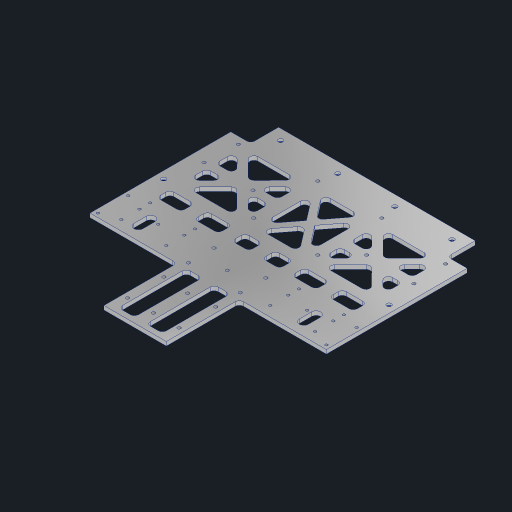
# Autodesk Inventor part: base
Saved by Autodesk Inventor 2023 (Build 270158000, 158)
## iProperties
Created: 2024-04-10
Part Number: base
Material: Aluminum 6061
Document SubType Name: Modeling
Designer: szymo
Density: 2.7 g/cm^3
Appearance: Aluminum - Flat
Mass: 138.037 g
Surface Area: 408.524 cm^2
Volume: 51.1249 cm^3
Author: szymo
Autodesk Inventor part; units mm, degrees
ref_plane "YZ Plane" through (0, 0, 0) normal (1, 0, 0) x (0, 1, 0)
ref_plane "XZ Plane" through (0, 0, 0) normal (0, 1, 0) x (-1, 0, 0)
ref_plane "XY Plane" through (0, 0, 0) normal (0, 0, 1) x (1, 0, 0)
sketch "Sketch2" plane through (0, 0, 0) normal (0, 1, 0) x (-1, 0, 0)
  line L0 (-89, 99) -> (89, 99)
  line L1 (89, 99) -> (89, -99)
  line L2 (89, -99) -> (-89, -99)
  line L3 (-89, -99) -> (-89, 99)
  line L4 (-89, 99) -> (89, -99) construction
  line L5 (89, 99) -> (-89, -99) construction
  line L6 (-89, 99) -> (89, 99)
  line L7 (89, 99) -> (89, -85)
  line L8 (89, -85) -> (-89, -85)
  line L9 (-89, -85) -> (-89, 99)
  line L10 (-4.5, 99) -> (-89, 99)
  line L11 (-89, 99) -> (-89, 42)
  line L12 (-89, 42) -> (-4.5, 42)
  line L13 (-4.5, 42) -> (-4.5, 99)
  line L14 (4.5, 99) -> (89, 99)
  line L15 (89, 99) -> (89, 42)
  line L16 (89, 42) -> (4.5, 42)
  line L17 (4.5, 42) -> (4.5, 99)
  line L18 (22.5, 77.5) -> (22.5, 66.5) projected
  line L19 (16.5, 66.5) -> (16.5, 77.5) projected
  line L20 (-22.5, 66.5) -> (-22.5, 77.5) projected
  line L21 (-16.5, 77.5) -> (-16.5, 66.5) projected
  line L22 (-23.5, 99) -> (-16.5, 99)
  line L23 (-16.5, 99) -> (-16.5, 42)
  line L24 (-16.5, 42) -> (-23.5, 42)
  line L25 (-23.5, 42) -> (-23.5, 99)
  line L26 (16.5, 99) -> (23.5, 99)
  line L27 (23.5, 99) -> (23.5, 42)
  line L28 (23.5, 42) -> (16.5, 42)
  line L29 (16.5, 42) -> (16.5, 99)
  line L30 (-89, 99) -> (89, 99)
  line L31 (89, 99) -> (89, 97)
  line L32 (89, 97) -> (-89, 97)
  line L33 (-89, 97) -> (-89, 99)
  line L34 (89, -85) -> (74, -85)
  line L35 (74, -85) -> (74, -64)
  line L36 (74, -64) -> (89, -64)
  line L37 (89, -64) -> (89, -85)
  line L38 (-89, -85) -> (-74, -85)
  line L39 (-74, -85) -> (-74, -64)
  line L40 (-74, -64) -> (-89, -64)
  line L41 (-89, -64) -> (-89, -85)
  line L42 (16.5, 97) -> (-16.5, 97)
  line L43 (-16.5, 97) -> (-16.5, 93)
  line L44 (-16.5, 93) -> (16.5, 93)
  line L45 (16.5, 93) -> (16.5, 97)
  line L46 (-84.4, -75) -> (-84.4, -71.5) projected
  line L47 (-84.4, -71.5) -> (-87, -71.5) projected
  line L48 (-87, -71.5) -> (-87, -75) projected
  line L49 (-87, -75) -> (-84.4, -75) projected
  line L50 (-79.6, -75) -> (-77, -75) projected
  line L51 (-77, -75) -> (-77, -71.5) projected
  line L52 (-77, -71.5) -> (-79.6, -71.5) projected
  line L53 (-79.6, -71.5) -> (-79.6, -75) projected
  line L54 (-75, -78) -> (-89, -78) projected
  line L55 (-89, -78) -> (-89, -63) projected
  line L56 (-89, -63) -> (-75, -63) projected
  line L57 (-75, -63) -> (-75, -78) projected
  circle A0 centre (-80.45, -67.25) radius 1.25 projected
  point P0 (0, 0)
  point P1 (4.5, 99)
  point P2 (-4.5, 99)
  point P3 (-89, 42)
  point P4 (89, 42)
  point P5 (4.5, 97)
  point P6 (-4.5, 97)
  point P7 (-16.5, 97)
  point P8 (-23.5, 97)
  point P9 (23.5, 97)
  point P10 (16.5, 98)
  point P11 (-4.5, 93)
  point P12 (4.5, 93)
  point P13 (16.5, 93)
  dimension "d8" = 178
  dimension "d9" = 198
  dimension "d10" = 14
  dimension "d11" = 84.5
  dimension "d13" = 84.5
  dimension "d17" = 9
  dimension "d18" = 2
  dimension "d19" = 15
  dimension "d20" = 21
  dimension "d21" = 15
  dimension "d22" = 21
  dimension "d75" = 55
  dimension "d76" = 55
  dimension "d77" = 7
  dimension "d78" = 7
  dimension "d79" = 4
  constraints: 84 end point, 20 parallel, 10 horizontal, 10 perpendicular, 10 point on line, 2 collinear, 2 midpoint, 5 other
  measures "d8" distance of L1.end L2.end
  measures "d9" distance of L0.end L1.end
  measures "d10" distance between parallel lines of L8 L2
  measures "d11" distance of L12.end L11.end
  measures "d13" distance of L15.end L16.end
  measures "d17" distance between parallel lines of L13 L17
  measures "d18" distance of L30.end L31.end
  measures "d19" distance of L35.end L36.end
  measures "d20" distance of L34.end L35.end
  measures "d21" distance of L40.end L39.end
  measures "d22" distance of L39.end L38.end
  measures "d75" distance between parallel lines of L32 L12
  measures "d76" distance between parallel lines of L32 L16
  measures "d77" distance between parallel lines of L23 L25
  measures "d78" distance between parallel lines of L27 L29
  measures "d79" distance of L43.end L42.end
extrude "Extrusion2" add sketch "Sketch2" along normal blind 3 contours L32 L23 L21 L12 L25 | L12 L13 L44 L17 L16 L1 L36 L35 L8 L39 L40 L57 L56 L3 | L32 L13 L44 L23 | L56 L57 L40 L3 | L32 L17 L44 L13 | L32 L29 L44 L17 | L32 L27 L16 L29 L19
fillet "Fillet5" radius 3 12 edges at (-16.5, 1.5, 42) (-4.5, 1.5, 42) (-23.5, 1.5, 42) (16.5, 1.5, 42) (-16.5, 1.5, 93) (-4.5, 1.5, 93) (4.5, 1.5, 93) (16.5, 1.5, 93) (4.5, 1.5, 42) (23.5, 1.5, 42) (74, 1.5, -64) (-74, 1.5, -64)
sketch "Sketch7" plane through (0, 3, 0) normal (0, 1, 0) x (1, 0, 0)
  circle A0 centre (78, 58.6725) radius 1.8 projected
  circle A1 centre (79, 33.8889) radius 1.8 projected
  circle A2 centre (42.5, 34.7802) radius 1.8 projected
  circle A3 centre (24.1, 64.6) radius 1.6 projected
  circle A4 centre (24.1, 16.4) radius 1.6 projected
  circle A5 centre (-24.1, 16.4) radius 1.6 projected
  circle A6 centre (-24.1, 64.6) radius 1.6 projected
  circle A7 centre (-42.5, 34.2745) radius 1.8 projected
  circle A8 centre (-79, 33.8889) radius 1.8 projected
  circle A9 centre (-78, 58.6725) radius 1.8 projected
  circle A10 centre (19.5, -18.05) radius 1.8 projected
  circle A11 centre (19.5, -37.375) radius 1.8 projected
  circle A12 centre (19.5, -55.8) radius 1.8 projected
  circle A13 centre (19.4231, -83.3077) radius 1.8 projected
  circle A14 centre (0, -83.2) radius 1.8 projected
  circle A15 centre (-19.4231, -83.3077) radius 1.8 projected
  circle A16 centre (-19.5, -55.8) radius 1.8 projected
  circle A17 centre (0, -57.55) radius 1.8 projected
  circle A18 centre (0, -27.625) radius 1.8 projected
  circle A19 centre (-19.5, -37.375) radius 1.8 projected
  circle A20 centre (-19.5, -18.05) radius 1.8 projected
  point P0 (0, 0)
  point P1 (-19.5, -83.2)
  constraints: 20 coincident
hole "Hole3" at (19.4231, 3, 83.3077) at (0, 3, 83.2) at (-19.5, 3, 83.2) at (19.5, 3, 55.8) at (0, 3, 57.55) at (-19.5, 3, 55.8) at (-19.5, 3, 37.375) at (-19.5, 3, 18.05) at (0, 3, 27.625) at (19.5, 3, 37.375) at (19.5, 3, 18.05) at (79, 3, -33.8889) at (78, 3, -58.6725) at (42.5, 3, -34.7802) at (24.1, 3, -16.4) at (-24.1, 3, -16.4) at (-24.1, 3, -64.6) at (24.1, 3, -64.6) at (-42.5, 3, -34.2745) at (-78, 3, -58.6725) at (-79, 3, -33.8889) direction (0, -1, 0) diameter 2.459 end through all thread size "M3x0.5" class "6H" standard "ISO Metric profile"
sketch "Sketch8" plane through (0, 3, 0) normal (0, 1, 0) x (1, 0, 0)
  circle A0 centre (72.95, -34.475) radius 1.45 projected
  circle A1 centre (72.95, -20.775) radius 1.45 projected
  circle A2 centre (39.125, -20.8375) radius 1.55 projected
  circle A3 centre (39.125, -34.4125) radius 1.55 projected
  circle A4 centre (-39.125, -20.8375) radius 1.55 projected
  circle A5 centre (-39.125, -34.4125) radius 1.55 projected
  circle A6 centre (-72.95, -34.475) radius 1.45 projected
  circle A7 centre (-72.95, -20.775) radius 1.45 projected
  circle A8 centre (86, -16.25) radius 2.3 projected
  circle A9 centre (86, -39) radius 2.3 projected
  circle A10 centre (86, 32.8889) radius 2.3 projected
  line L0 (89, -42) -> (83, -42) projected
  line L1 (89, 35.8889) -> (89, -42) projected
  line L2 (89, 35.8889) -> (83, 35.8889) projected
  line L3 (83, 29.8889) -> (83, 35.8889) projected
  line L4 (83, 29.8889) -> (87.4, 29.8889) projected
  line L5 (87.4, 29.8889) -> (87.4, 14.7889) projected
  line L6 (87.4, 14.7889) -> (79.4, 14.7889) projected
  line L7 (79.4, 2.7889) -> (79.4, 14.7889) projected
  line L8 (86, 2.7889) -> (79.4, 2.7889) projected
  line L9 (86, -13.25) -> (86, 2.7889) projected
  line L10 (86, -13.25) -> (83, -13.25) projected
  line L11 (83, -13.25) -> (83, -19.25) projected
  line L12 (83, -19.25) -> (86, -19.25) projected
  line L13 (86, -36) -> (86, -19.25) projected
  line L14 (86, -36) -> (83, -36) projected
  line L15 (83, -36) -> (83, -42) projected
  circle A11 centre (83.4, 10.7889) radius 2.6 projected
  circle A12 centre (-86, -39) radius 2.3 projected
  circle A13 centre (-86, -16.25) radius 2.3 projected
  line L16 (-86, -13.25) -> (-86, -0.1111) projected
  line L17 (-79.4, -0.1111) -> (-86, -0.1111) projected
  line L18 (-79.4, 11.8889) -> (-79.4, -0.1111) projected
  line L19 (-86, 11.8889) -> (-79.4, 11.8889) projected
  line L20 (-86, 11.8889) -> (-86, 29.8889) projected
  line L21 (-86, 29.8889) -> (-83, 29.8889) projected
  line L22 (-83, 29.8889) -> (-83, 35.8889) projected
  line L23 (-89, 35.8889) -> (-83, 35.8889) projected
  line L24 (-89, 35.8889) -> (-89, -42) projected
  line L25 (-89, -42) -> (-83, -42) projected
  line L26 (-83, -42) -> (-83, -36) projected
  line L27 (-83, -36) -> (-86, -36) projected
  line L28 (-86, -36) -> (-86, -19.25) projected
  line L29 (-86, -19.25) -> (-83, -19.25) projected
  line L30 (-83, -19.25) -> (-83, -13.25) projected
  line L31 (-83, -13.25) -> (-86, -13.25) projected
  circle A14 centre (-86, 32.8889) radius 2.3 projected
  circle A15 centre (-83.4, 7.8889) radius 2.6 projected
  line L32 (72.95, -34.475) -> (39.125, -12.8375)
  line L33 (72.95, -12.775) -> (39.125, -34.4125)
  line L34 (-39.125, -34.4125) -> (-72.95, -12.775)
  line L35 (-39.125, -12.8375) -> (-72.95, -34.4125)
  point P0 (0, 0)
  point P1 (56.0375, -23.5937)
  point P2 (-56.0375, -23.625)
  dimension "d90" = 8
  dimension "d91" = 8
  dimension "d92" = 8
  dimension "d93" = 8
  constraints: 12 coincident, 8 end point, 2 midpoint
  measures "d90" distance of A1.centre L33.start
  measures "d91" distance of L32.end A2.centre
  measures "d92" distance of point (-39.125, -20.837) L35.start
  measures "d93" distance of A7.centre L34.end
hole "Hole4" at (72.95, 3, 34.475) at (72.95, 3, 20.775) at (39.125, 3, 20.8375) at (39.125, 3, 34.4125) at (86, 3, 39) at (86, 3, 16.25) at (-86, 3, 39) at (-86, 3, 16.25) at (-72.95, 3, 20.775) at (-72.95, 3, 34.475) at (-39.125, 3, 34.4125) at (-39.125, 3, 20.8375) at (72.95, 3, 12.775) at (39.125, 3, 12.8375) at (-39.125, 3, 12.8375) at (-72.95, 3, 12.775) at (56.0375, 3, 23.5937) at (-56.0375, 3, 23.625) direction (0, -1, 0) diameter 2.013 end through all thread size "M2.5x0.45" class "6H" standard "ISO Metric profile"
sketch "Sketch9" plane through (0, 0, 0) normal (0, -1, 0) x (1, 0, 0)
  circle A0 centre (64.5, -77) radius 1.2295 projected
  circle A1 centre (21.5, -77) radius 1.2295 projected
  circle A2 centre (-21.5, -77) radius 1.2295 projected
  circle A3 centre (-64.5, -77) radius 1.2295 projected
  circle A4 centre (-83.4, -7.8889) radius 2.6 projected
  circle A5 centre (83.4, -10.7889) radius 2.6 projected
  point P0 (0, 0)
  constraints: 6 coincident
hole "Hole5" at (-83.4, 0, -7.8889) at (83.4, 0, -10.7889) at (64.5, 0, -77) at (21.5, 0, -77) at (-21.5, 0, -77) at (-64.5, 0, -77) direction (0, 1, 0) diameter 3.6 end through all countersink diameter 6.6 countersink angle 90 clearance for "Countersunk Flat Head Screw ISO 2009/7046" size "M3" standard "ISO"
sketch "Sketch10" plane through (0, 0, 0) normal (0, -1, 0) x (1, 0, 0)
  line L0 (-23.5, -30) -> (-22.5, -31)
  line L1 (-27.5, -30) -> (-23.5, -30)
  line L2 (-27.5, -13) -> (-27.5, -30)
  line L3 (-17.5, -13) -> (-27.5, -13)
  line L4 (-17.5, -19) -> (-17.5, -13)
  line L5 (-15.5, -21) -> (-17.5, -19)
  line L6 (16.5, -21) -> (-15.5, -21)
  line L7 (18.5, -19) -> (16.5, -21)
  line L8 (18.5, -13) -> (18.5, -19)
  line L9 (27.5, -13) -> (18.5, -13)
  line L10 (27.5, -20) -> (27.5, -13)
  line L11 (23.5, -20) -> (27.5, -20)
  line L12 (22.5, -21) -> (23.5, -20)
  line L13 (22.5, -43) -> (22.5, -21)
  line L14 (23.5, -44) -> (22.5, -43)
  line L15 (27.5, -44) -> (23.5, -44)
  line L16 (27.5, -68) -> (27.5, -44)
  line L17 (-27.5, -68) -> (27.5, -68)
  line L18 (-27.5, -44) -> (-27.5, -68)
  line L19 (-23.5, -44) -> (-27.5, -44)
  line L20 (-22.5, -43) -> (-23.5, -44)
  line L21 (-22.5, -31) -> (-22.5, -43)
  circle A0 centre (26.5, -60.54) radius 0.325
  circle A1 centre (26.5, -59.27) radius 0.325
  circle A2 centre (-24.1, -64.6) radius 1.6
  circle A3 centre (26.5, -58) radius 0.325
  circle A4 centre (24.1, -64.6) radius 1.6
  circle A5 centre (26.5, -56.73) radius 0.325
  circle A6 centre (26.5, -53) radius 0.325
  circle A7 centre (26.5, -54.27) radius 0.325
  circle A8 centre (26.5, -51.73) radius 0.325
  circle A9 centre (26.5, -50.46) radius 0.325
  circle A10 centre (24.1, -16.4) radius 1.6
  circle A11 centre (-26.5, -56.73) radius 0.325
  circle A12 centre (-26.5, -54.27) radius 0.325
  circle A13 centre (-26.5, -60.54) radius 0.325
  circle A14 centre (-26.5, -58) radius 0.325
  circle A15 centre (-26.5, -59.27) radius 0.325
  circle A16 centre (-25, -26.77) radius 0.45
  circle A17 centre (-24.1, -16.4) radius 1.6
  circle A18 centre (-25, -24.23) radius 0.45
  circle A19 centre (-26.5, -53) radius 0.325
  circle A20 centre (-26.5, -50.46) radius 0.325
  circle A21 centre (-26.5, -51.73) radius 0.325
  circle A22 centre (21.5, -77) radius 1.2295
  circle A23 centre (-64.5, -77) radius 1.2295
  circle A24 centre (-21.5, -77) radius 1.2295
  circle A25 centre (64.5, -77) radius 1.2295
  line L22 (-72, -79) -> (-72, -70)
  line L23 (-72, -70) -> (-57, -70)
  line L24 (-57, -70) -> (-57, -79)
  arc A26 (-57, -79) -> (-55, -81) centre (-55, -79) ccw
  line L25 (-55, -81) -> (-31, -81)
  arc A27 (-31, -81) -> (-29, -79) centre (-31, -79) ccw
  line L26 (-29, -79) -> (-29, -70)
  line L27 (-29, -70) -> (-14, -70)
  line L28 (-14, -70) -> (-14, -79)
  arc A28 (-14, -79) -> (-12, -81) centre (-12, -79) ccw
  line L29 (-12, -81) -> (12, -81)
  arc A29 (12, -81) -> (14, -79) centre (12, -79) ccw
  line L30 (14, -79) -> (14, -70)
  line L31 (14, -70) -> (29, -70)
  line L32 (29, -70) -> (29, -79)
  arc A30 (29, -79) -> (31, -81) centre (31, -79) ccw
  line L33 (31, -81) -> (55, -81)
  arc A31 (55, -81) -> (57, -79) centre (55, -79) ccw
  line L34 (57, -79) -> (57, -70)
  line L35 (57, -70) -> (72, -70)
  line L36 (72, -70) -> (72, -79)
  arc A32 (72, -79) -> (74, -81) centre (74, -79) ccw
  line L37 (74, -81) -> (89, -81)
  line L38 (89, -85) -> (89, -81)
  line L39 (-89, -85) -> (89, -85)
  line L40 (-89, -85) -> (-89, -81)
  line L41 (-89, -81) -> (-74, -81)
  arc A33 (-74, -81) -> (-72, -79) centre (-74, -79) ccw
  line L42 (-89, -99) -> (-89, -85)
  line L43 (-89, -85) -> (89, -85)
  line L44 (89, -99) -> (89, -85)
  line L45 (-89, -99) -> (89, -99)
  circle A34 centre (78, -58.6725) radius 1.8
  circle A35 centre (79, -33.8889) radius 1.8
  circle A36 centre (83.4, -10.7889) radius 2.6
  circle A37 centre (80.5, -70.5) radius 1.75
  circle A38 centre (42.5, -34.7802) radius 1.8
  spline S0 degree 2 poles (89, 38.051) (88.5208, 39.25) (89, 40.449) knots 0 0 0 1 1 1 weights 1 1.090909 1
  line L46 (89, 42) -> (89, 40.449)
  line L47 (89, 42) -> (86, 42)
  line L48 (86, -2.7889) -> (86, 42)
  line L49 (79.4, -2.7889) -> (86, -2.7889)
  line L50 (79.4, -14.7889) -> (79.4, -2.7889)
  line L51 (86, -14.7889) -> (79.4, -14.7889)
  line L52 (86, -16.7889) -> (86, -14.7889)
  line L53 (86, -27.8889) -> (86, -16.7889)
  line L54 (86, -29.8889) -> (86, -27.8889)
  line L55 (39, -29.8889) -> (86, -29.8889)
  line L56 (39, -39.6715) -> (39, -29.8889)
  line L57 (46, -39.6715) -> (39, -39.6715)
  line L58 (46, -41.6649) -> (46, -39.6715)
  line L59 (46, -41.6649) -> (77.5308, -41.6649)
  ellipse E0 centre (76.799, -27.2986) end of major axis (76.7969, -11.6653) minor radius 1.851 (76.801, -42.9318) -> (77.5308, -41.6649) ccw
  line L60 (76.801, -42.9318) -> (67, -42.9318)
  line L61 (67, -53.3451) -> (67, -42.9318)
  line L62 (73, -53.3451) -> (67, -53.3451)
  line L63 (73, -75) -> (73, -53.3451)
  line L64 (83, -75) -> (73, -75)
  line L65 (83, -81) -> (83, -75)
  line L66 (89, -81) -> (83, -81)
  line L67 (89, 14.801) -> (89, -81)
  spline S1 degree 2 poles (89, 14.801) (88.5208, 16) (89, 17.199) knots 0 0 0 1 1 1 weights 1 1.090909 1
  line L68 (89, 38.051) -> (89, 17.199)
  circle A39 centre (-42.5, -34.2745) radius 1.8
  line L69 (-86, 0.1111) -> (-86, 42)
  line L70 (-89, 42) -> (-86, 42)
  line L71 (-89, 42) -> (-89, 38.75)
  line L72 (-89, 38.75) -> (-89, 13.5)
  line L73 (-89, 13.5) -> (-89, -81)
  line L74 (-89, -81) -> (-83, -81)
  line L75 (-83, -81) -> (-83, -75)
  line L76 (-83, -75) -> (-73, -75)
  line L77 (-73, -75) -> (-73, -53.3451)
  line L78 (-73, -53.3451) -> (-67, -53.3451)
  line L79 (-67, -53.3451) -> (-67, -42.9318)
  line L80 (-76.801, -42.9318) -> (-67, -42.9318)
  ellipse E1 centre (-76.799, -27.2986) end of major axis (-76.7969, -11.6653) minor radius 1.851 (-77.5308, -41.6649) -> (-76.801, -42.9318) ccw
  line L81 (-46, -41.6649) -> (-77.5308, -41.6649)
  line L82 (-46, -38.66) -> (-46, -41.6649)
  line L83 (-39, -38.66) -> (-46, -38.66)
  line L84 (-39, -29.8889) -> (-39, -38.66)
  line L85 (-52, -29.8889) -> (-39, -29.8889)
  line L86 (-52, -34.8889) -> (-52, -29.8889)
  line L87 (-75, -34.8889) -> (-52, -34.8889)
  line L88 (-75, -34.8889) -> (-75, -29.8889)
  line L89 (-86, -29.8889) -> (-75, -29.8889)
  line L90 (-86, -29.8889) -> (-86, -11.8889)
  line L91 (-79.4, -11.8889) -> (-86, -11.8889)
  line L92 (-79.4, 0.1111) -> (-79.4, -11.8889)
  line L93 (-86, 0.1111) -> (-79.4, 0.1111)
  circle A40 centre (-83.5, -70.5) radius 1.75
  circle A41 centre (-79, -33.8889) radius 1.8
  circle A42 centre (-83.4, -7.8889) radius 2.6
  circle A43 centre (-78, -58.6725) radius 1.8
  line L94 (-47.199, -41.6649) -> (-47.5424, -51.3902)
  line L95 (-76.801, -41.6649) -> (-47.199, -41.6649)
  line L96 (-76.4576, -51.3902) -> (-76.801, -41.6649)
  line L97 (-76.4545, -51.3901) -> (-76.4576, -51.3902)
  line L98 (-47.5455, -51.3901) -> (-76.4545, -51.3901)
  line L99 (-47.5424, -51.3902) -> (-47.5455, -51.3901)
  line L100 (47.199, -41.6649) -> (47.5424, -51.3902)
  line L101 (47.5424, -51.3902) -> (47.5455, -51.3901)
  line L102 (47.5455, -51.3901) -> (76.4545, -51.3901)
  line L103 (76.4545, -51.3901) -> (76.4576, -51.3902)
  line L104 (76.4576, -51.3902) -> (76.801, -41.6649)
  line L105 (76.801, -41.6649) -> (47.199, -41.6649)
  circle A44 centre (72.95, 34.475) radius 1.45
  circle A45 centre (72.95, 20.775) radius 1.45
  circle A46 centre (39.125, 34.4125) radius 1.55
  circle A47 centre (39.125, 20.8375) radius 1.55
  spline S2 degree 3 poles (65.7, 23.025) (65.7, 22.8819) (65.6837, 22.6312) (65.6334, 22.3458) (65.5819, 22.1333) (65.5405, 21.9923) (65.48, 21.8179) (65.4239, 21.6792) (65.3456, 21.5106) (65.2769, 21.3802) (65.184, 21.2227) (65.1043, 21.1011) (64.9982, 20.9549) (64.9083, 20.8425) (64.7662, 20.6811) (64.615, 20.5299) (64.3941, 20.3423) (64.2146, 20.2128) (64.0241, 20.0935) (63.8917, 20.0193) (63.7367, 19.9424) (63.63, 19.8951) (63.5206, 19.8513) (63.4473, 19.8241) (63.3368, 19.7865) (63.2255, 19.7528) (63.02, 19.6999) (62.7939, 19.6576) (62.4526, 19.6224) (62.1474, 19.6224) (61.8061, 19.6576) (61.58, 19.6999) (61.3745, 19.7528) (61.2632, 19.7865) (61.1527, 19.8241) (61.0794, 19.8513) (60.97, 19.8951) (60.8633, 19.9424) (60.7083, 20.0193) (60.5759, 20.0935) (60.3854, 20.2128) (60.2059, 20.3423) (59.985, 20.5299) (59.8338, 20.6811) (59.6917, 20.8425) (59.6018, 20.9549) (59.4957, 21.1011) (59.416, 21.2227) (59.3231, 21.3802) (59.2544, 21.5106) (59.1761, 21.6792) (59.12, 21.8179) (59.0595, 21.9923) (59.0181, 22.1333) (58.9666, 22.3458) (58.9163, 22.6312) (58.9, 22.8819) (58.9, 23.025) knots 0.368505 0.368505 0.368505 0.368505 0.400174 0.423925 0.431842 0.447677 0.455594 0.471428 0.479345 0.49518 0.503097 0.518931 0.526849 0.542683 0.5506 0.574352 0.590186 0.613938 0.621855 0.637689 0.645607 0.657482 0.661441 0.669358 0.673317 0.685193 0.69311 0.716861 0.732696 0.764365 0.780199 0.803951 0.811868 0.823744 0.827702 0.835619 0.839578 0.851454 0.859371 0.875205 0.883123 0.906874 0.922709 0.94646 0.954377 0.970212 0.978129 0.993963 1.00188 1.017715 1.025632 1.041466 1.049384 1.065218 1.073135 1.096887 1.128556 1.128556 1.128556 1.128556
  line L106 (58.9, 23.025) -> (58.9, 32.225)
  spline S3 degree 3 poles (58.9, 32.225) (58.9, 32.3681) (58.9163, 32.6188) (58.9666, 32.9042) (59.0181, 33.1167) (59.0595, 33.2577) (59.12, 33.4321) (59.1761, 33.5708) (59.2544, 33.7394) (59.3231, 33.8698) (59.416, 34.0273) (59.4957, 34.1489) (59.6018, 34.2951) (59.6917, 34.4075) (59.8338, 34.5689) (59.985, 34.7201) (60.2059, 34.9077) (60.3854, 35.0372) (60.5759, 35.1565) (60.7083, 35.2307) (60.8633, 35.3076) (60.97, 35.3549) (61.0794, 35.3987) (61.1527, 35.4259) (61.2632, 35.4635) (61.3745, 35.4972) (61.58, 35.5501) (61.8061, 35.5924) (62.1474, 35.6276) (62.4526, 35.6276) (62.7939, 35.5924) (63.02, 35.5501) (63.2255, 35.4972) (63.3368, 35.4635) (63.4473, 35.4259) (63.5206, 35.3987) (63.63, 35.3549) (63.7367, 35.3076) (63.8917, 35.2307) (64.0241, 35.1565) (64.2146, 35.0372) (64.3941, 34.9077) (64.615, 34.7201) (64.7662, 34.5689) (64.9083, 34.4075) (64.9982, 34.2951) (65.1043, 34.1489) (65.184, 34.0273) (65.2769, 33.8698) (65.3456, 33.7394) (65.4239, 33.5708) (65.48, 33.4321) (65.5405, 33.2577) (65.5819, 33.1167) (65.6334, 32.9042) (65.6837, 32.6188) (65.7, 32.3681) (65.7, 32.225) knots -0.380025 -0.380025 -0.380025 -0.380025 -0.348357 -0.324605 -0.316688 -0.300853 -0.292936 -0.277102 -0.269185 -0.25335 -0.245433 -0.229599 -0.221682 -0.205847 -0.19793 -0.174178 -0.158344 -0.134592 -0.126675 -0.110841 -0.102924 -0.091048 -0.087089 -0.079172 -0.075213 -0.063338 -0.05542 -0.031669 -0.015834 0.015834 0.031669 0.05542 0.063338 0.075213 0.079172 0.087089 0.091048 0.102924 0.110841 0.126675 0.134592 0.158344 0.174178 0.19793 0.205847 0.221682 0.229599 0.245433 0.25335 0.269185 0.277102 0.292936 0.300853 0.316688 0.324605 0.348357 0.380025 0.380025 0.380025 0.380025
  line L107 (65.7, 32.225) -> (65.7, 23.025)
  line L108 (27.2, 42) -> (86, 42)
  line L109 (27.2, 13.25) -> (27.2, 42)
  line L110 (27.2, 13.25) -> (86, 13.25)
  line L111 (86, 42) -> (86, 13.25)
  circle A48 centre (-72.95, 34.475) radius 1.45
  circle A49 centre (-72.95, 20.775) radius 1.45
  circle A50 centre (-39.125, 34.4125) radius 1.55
  circle A51 centre (-39.125, 20.8375) radius 1.55
  spline S4 degree 3 poles (-65.7, 23.025) (-65.7, 22.8819) (-65.6837, 22.6312) (-65.6334, 22.3458) (-65.5819, 22.1333) (-65.5405, 21.9923) (-65.48, 21.8179) (-65.4239, 21.6792) (-65.3456, 21.5106) (-65.2769, 21.3802) (-65.184, 21.2227) (-65.1043, 21.1011) (-64.9982, 20.9549) (-64.9083, 20.8425) (-64.7662, 20.6811) (-64.615, 20.5299) (-64.3941, 20.3423) (-64.2146, 20.2128) (-64.0241, 20.0935) (-63.8917, 20.0193) (-63.7367, 19.9424) (-63.63, 19.8951) (-63.5206, 19.8513) (-63.4473, 19.8241) (-63.3368, 19.7865) (-63.2255, 19.7528) (-63.02, 19.6999) (-62.7939, 19.6576) (-62.4526, 19.6224) (-62.1474, 19.6224) (-61.8061, 19.6576) (-61.58, 19.6999) (-61.3745, 19.7528) (-61.2632, 19.7865) (-61.1527, 19.8241) (-61.0794, 19.8513) (-60.97, 19.8951) (-60.8633, 19.9424) (-60.7083, 20.0193) (-60.5759, 20.0935) (-60.3854, 20.2128) (-60.2059, 20.3423) (-59.985, 20.5299) (-59.8338, 20.6811) (-59.6917, 20.8425) (-59.6018, 20.9549) (-59.4957, 21.1011) (-59.416, 21.2227) (-59.3231, 21.3802) (-59.2544, 21.5106) (-59.1761, 21.6792) (-59.12, 21.8179) (-59.0595, 21.9923) (-59.0181, 22.1333) (-58.9666, 22.3458) (-58.9163, 22.6312) (-58.9, 22.8819) (-58.9, 23.025) knots 0.368505 0.368505 0.368505 0.368505 0.400174 0.423925 0.431842 0.447677 0.455594 0.471428 0.479345 0.49518 0.503097 0.518931 0.526849 0.542683 0.5506 0.574352 0.590186 0.613938 0.621855 0.637689 0.645607 0.657482 0.661441 0.669358 0.673317 0.685193 0.69311 0.716861 0.732696 0.764365 0.780199 0.803951 0.811868 0.823744 0.827702 0.835619 0.839578 0.851454 0.859371 0.875205 0.883123 0.906874 0.922709 0.94646 0.954377 0.970212 0.978129 0.993963 1.00188 1.017715 1.025632 1.041466 1.049384 1.065218 1.073135 1.096887 1.128556 1.128556 1.128556 1.128556
  line L112 (-65.7, 32.225) -> (-65.7, 23.025)
  spline S5 degree 3 poles (-58.9, 32.225) (-58.9, 32.3681) (-58.9163, 32.6188) (-58.9666, 32.9042) (-59.0181, 33.1167) (-59.0595, 33.2577) (-59.12, 33.4321) (-59.1761, 33.5708) (-59.2544, 33.7394) (-59.3231, 33.8698) (-59.416, 34.0273) (-59.4957, 34.1489) (-59.6018, 34.2951) (-59.6917, 34.4075) (-59.8338, 34.5689) (-59.985, 34.7201) (-60.2059, 34.9077) (-60.3854, 35.0372) (-60.5759, 35.1565) (-60.7083, 35.2307) (-60.8633, 35.3076) (-60.97, 35.3549) (-61.0794, 35.3987) (-61.1527, 35.4259) (-61.2632, 35.4635) (-61.3745, 35.4972) (-61.58, 35.5501) (-61.8061, 35.5924) (-62.1474, 35.6276) (-62.4526, 35.6276) (-62.7939, 35.5924) (-63.02, 35.5501) (-63.2255, 35.4972) (-63.3368, 35.4635) (-63.4473, 35.4259) (-63.5206, 35.3987) (-63.63, 35.3549) (-63.7367, 35.3076) (-63.8917, 35.2307) (-64.0241, 35.1565) (-64.2146, 35.0372) (-64.3941, 34.9077) (-64.615, 34.7201) (-64.7662, 34.5689) (-64.9083, 34.4075) (-64.9982, 34.2951) (-65.1043, 34.1489) (-65.184, 34.0273) (-65.2769, 33.8698) (-65.3456, 33.7394) (-65.4239, 33.5708) (-65.48, 33.4321) (-65.5405, 33.2577) (-65.5819, 33.1167) (-65.6334, 32.9042) (-65.6837, 32.6188) (-65.7, 32.3681) (-65.7, 32.225) knots -0.380025 -0.380025 -0.380025 -0.380025 -0.348357 -0.324605 -0.316688 -0.300853 -0.292936 -0.277102 -0.269185 -0.25335 -0.245433 -0.229599 -0.221682 -0.205847 -0.19793 -0.174178 -0.158344 -0.134592 -0.126675 -0.110841 -0.102924 -0.091048 -0.087089 -0.079172 -0.075213 -0.063338 -0.05542 -0.031669 -0.015834 0.015834 0.031669 0.05542 0.063338 0.075213 0.079172 0.087089 0.091048 0.102924 0.110841 0.126675 0.134592 0.158344 0.174178 0.19793 0.205847 0.221682 0.229599 0.245433 0.25335 0.269185 0.277102 0.292936 0.300853 0.316688 0.324605 0.348357 0.380025 0.380025 0.380025 0.380025
  line L113 (-58.9, 23.025) -> (-58.9, 32.225)
  line L114 (-27.2, 42) -> (-86, 42)
  line L115 (-86, 42) -> (-86, 13.25)
  line L116 (-27.2, 13.25) -> (-86, 13.25)
  line L117 (-27.2, 13.25) -> (-27.2, 42)
  line L118 (-22.5, 14.25) -> (-16.5, 14.25)
  line L119 (-16.5, 97) -> (-16.5, 14.25)
  line L120 (-22.5, 97) -> (-16.5, 97)
  line L121 (-22.5, 14.25) -> (-22.5, 97)
  circle A52 centre (-19.5, 55.8) radius 1.8
  circle A53 centre (-19.5, 18.05) radius 1.8
  circle A54 centre (-19.5, 37.375) radius 1.8
  circle A55 centre (-19.4231, 83.3077) radius 1.8
  circle A56 centre (0, 57.55) radius 1.8
  circle A57 centre (0, 27.625) radius 1.8
  circle A58 centre (0, 83.2) radius 1.8
  line L122 (-4.5, 14.25) -> (-4.5, 97)
  line L123 (4.5, 14.25) -> (-4.5, 14.25)
  line L124 (4.5, 97) -> (4.5, 14.25)
  line L125 (-4.5, 97) -> (4.5, 97)
  line L126 (16.5, 14.25) -> (22.5, 14.25)
  line L127 (22.5, 97) -> (22.5, 14.25)
  line L128 (16.5, 97) -> (22.5, 97)
  line L129 (16.5, 14.25) -> (16.5, 97)
  circle A59 centre (19.4231, 83.3077) radius 1.8
  circle A60 centre (19.5, 37.375) radius 1.8
  circle A61 centre (19.5, 18.05) radius 1.8
  circle A62 centre (19.5, 55.8) radius 1.8
  line L130 (77.6433, -8.75) -> (11.6433, -8.75)
  line L131 (77.6433, 11.25) -> (77.6433, -8.75)
  line L132 (11.6433, 11.25) -> (77.6433, 11.25)
  line L133 (11.6433, -8.75) -> (11.6433, 11.25)
  line L134 (-77.0142, -3.75) -> (-9.0142, -3.75)
  line L135 (-9.0142, -3.75) -> (-9.0142, 11.25)
  line L136 (-9.0142, 11.25) -> (-77.0142, 11.25)
  line L137 (-77.0142, 11.25) -> (-77.0142, -3.75)
  circle A63 centre (-21.5, -77) radius 1.8
  circle A64 centre (64.5, -77) radius 1.8
  circle A65 centre (-83.4, -7.8889) radius 1.8
  circle A66 centre (83.4, -10.7889) radius 1.8
  circle A67 centre (21.5, -77) radius 1.8
  circle A68 centre (-64.5, -77) radius 1.8
  circle A69 centre (56.0375, 23.5937) radius 1.0065
  circle A70 centre (-39.125, 12.8375) radius 1.0065
  circle A71 centre (72.95, 12.775) radius 1.0065
  circle A72 centre (-39.125, 34.4125) radius 1.0065
  circle A73 centre (-72.95, 20.775) radius 1.0065
  circle A74 centre (-86, 39) radius 1.0065
  circle A75 centre (86, 39) radius 1.0065
  circle A76 centre (39.125, 20.8375) radius 1.0065
  circle A77 centre (72.95, 34.475) radius 1.0065
  circle A78 centre (72.95, 20.775) radius 1.0065
  circle A79 centre (39.125, 34.4125) radius 1.0065
  circle A80 centre (86, 16.25) radius 1.0065
  circle A81 centre (-86, 16.25) radius 1.0065
  circle A82 centre (-72.95, 34.475) radius 1.0065
  circle A83 centre (-39.125, 20.8375) radius 1.0065
  circle A84 centre (39.125, 12.8375) radius 1.0065
  circle A85 centre (-72.95, 12.775) radius 1.0065
  circle A86 centre (-56.0375, 23.625) radius 1.0065
  circle A87 centre (-78, -58.6725) radius 1.2295
  circle A88 centre (24.1, -64.6) radius 1.2295
  circle A89 centre (-24.1, -16.4) radius 1.2295
  circle A90 centre (42.5, -34.7802) radius 1.2295
  circle A91 centre (79, -33.8889) radius 1.2295
  circle A92 centre (19.5, 37.375) radius 1.2295
  circle A93 centre (-19.5, 18.05) radius 1.2295
  circle A94 centre (-19.5, 55.8) radius 1.2295
  circle A95 centre (19.5, 55.8) radius 1.2295
  circle A96 centre (0, 83.2) radius 1.2295
  circle A97 centre (19.4231, 83.3077) radius 1.2295
  circle A98 centre (-19.5, 83.2) radius 1.2295
  circle A99 centre (0, 57.55) radius 1.2295
  circle A100 centre (-19.5, 37.375) radius 1.2295
  circle A101 centre (0, 27.625) radius 1.2295
  circle A102 centre (19.5, 18.05) radius 1.2295
  circle A103 centre (78, -58.6725) radius 1.2295
  circle A104 centre (24.1, -16.4) radius 1.2295
  circle A105 centre (-24.1, -64.6) radius 1.2295
  circle A106 centre (-42.5, -34.2745) radius 1.2295
  circle A107 centre (-79, -33.8889) radius 1.2295
  line L138 (-16.5, 90) -> (-16.5, 45)
  arc A108 (-16.5, 45) -> (-13.5, 42) centre (-13.5, 45) ccw
  line L139 (-13.5, 42) -> (-7.5, 42)
  arc A109 (-7.5, 42) -> (-4.5, 45) centre (-7.5, 45) ccw
  line L140 (-4.5, 45) -> (-4.5, 90)
  arc A110 (-4.5, 90) -> (-7.5, 93) centre (-7.5, 90) ccw
  line L141 (-7.5, 93) -> (-13.5, 93)
  arc A111 (-13.5, 93) -> (-16.5, 90) centre (-13.5, 90) ccw
  line L142 (13.5, 93) -> (7.5, 93)
  arc A112 (7.5, 93) -> (4.5, 90) centre (7.5, 90) ccw
  line L143 (4.5, 90) -> (4.5, 45)
  arc A113 (4.5, 45) -> (7.5, 42) centre (7.5, 45) ccw
  line L144 (7.5, 42) -> (13.5, 42)
  arc A114 (13.5, 42) -> (16.5, 45) centre (13.5, 45) ccw
  line L145 (16.5, 45) -> (16.5, 90)
  arc A115 (16.5, 90) -> (13.5, 93) centre (13.5, 90) ccw
  line L146 (-23.5, 97) -> (23.5, 97)
  line L147 (23.5, 97) -> (23.5, 45)
  arc A116 (23.5, 45) -> (26.5, 42) centre (26.5, 45) ccw
  line L148 (26.5, 42) -> (89, 42)
  line L149 (89, 42) -> (89, -64)
  line L150 (89, -64) -> (77, -64)
  arc A117 (77, -64) -> (74, -67) centre (77, -67) ccw
  line L151 (74, -67) -> (74, -85)
  line L152 (74, -85) -> (-74, -85)
  line L153 (-74, -85) -> (-74, -67)
  arc A118 (-74, -67) -> (-77, -64) centre (-77, -67) ccw
  line L154 (-77, -64) -> (-89, -64)
  line L155 (-89, -64) -> (-89, 42)
  line L156 (-89, 42) -> (-26.5, 42)
  arc A119 (-26.5, 42) -> (-23.5, 45) centre (-26.5, 45) ccw
  line L157 (-23.5, 45) -> (-23.5, 97)
  line L158 (-74, -85) -> (74, -85)
  line L159 (74, -85) -> (74, -58)
  line L160 (74, -58) -> (-74, -58)
  line L161 (-74, -58) -> (-74, -85)
  line L162 (-24.1, -63) -> (24.1, -63) construction
  line L163 (-89, -64) -> (-74, -64)
  line L164 (-74, -64) -> (-74, 42)
  line L165 (-74, 42) -> (-89, 42)
  line L166 (-89, 42) -> (-89, -64)
  line L167 (89, -64) -> (74, -64)
  line L168 (74, -64) -> (74, 42)
  line L169 (74, 42) -> (89, 42)
  line L170 (89, 42) -> (89, -64)
  line L171 (-74, 42) -> (74, 42)
  line L172 (74, 42) -> (74, 6.7685)
  line L173 (-74, 6.7685) -> (-74, 42)
  circle A120 centre (-72.95, 12.775) radius 1.0065
  line L174 (-72.95, 11.7685) -> (72.95, 11.7685) construction
  line L175 (-27.5, 11.7685) -> (-17.5, 11.7685)
  line L176 (-17.5, 11.7685) -> (-17.5, -58)
  line L177 (-17.5, -58) -> (-27.5, -58)
  line L178 (-27.5, -58) -> (-27.5, 11.7685)
  line L179 (27.5, -58) -> (18.5, -58)
  line L180 (18.5, -58) -> (18.5, 11.7685)
  line L181 (18.5, 11.7685) -> (27.5, 11.7685)
  line L182 (27.5, 11.7685) -> (27.5, -58)
  line L183 (-27.5, 12.7685) -> (-27.5, 6.7685)
  line L184 (-27.5, 6.7685) -> (-74, 6.7685)
  line L185 (-74, 6.7685) -> (-74, 1.7685)
  line L186 (18.5, 12.7685) -> (18.5, 6.7685)
  line L187 (18.5, 6.7685) -> (-17.5, 6.7685)
  line L188 (-17.5, 6.7685) -> (-17.5, 1.7685)
  line L189 (74, 12.7685) -> (74, 6.7685)
  line L190 (74, 6.7685) -> (27.5, 6.7685)
  line L191 (27.5, 6.7685) -> (27.5, 1.7685)
  line L192 (-74, -3.2315) -> (-27.5, -3.2315)
  line L193 (-27.5, -3.2315) -> (-27.5, -11.2315)
  line L194 (-27.5, -11.2315) -> (-74, -11.2315)
  line L195 (-74, -11.2315) -> (-74, -3.2315)
  line L196 (-17.5, -3.2315) -> (18.5, -3.2315)
  line L197 (18.5, -3.2315) -> (18.5, -11.2315)
  line L198 (18.5, -11.2315) -> (-17.5, -11.2315)
  line L199 (-17.5, -11.2315) -> (-17.5, -3.2315)
  line L200 (27.5, -3.2315) -> (74, -3.2315)
  line L201 (74, -3.2315) -> (74, -11.2315)
  line L202 (74, -11.2315) -> (27.5, -11.2315)
  line L203 (27.5, -11.2315) -> (27.5, -3.2315)
  line L204 (-74, -11.2315) -> (-27.5, -58) construction
  line L205 (-27.5, -11.2315) -> (-74, -58) construction
  line L206 (-74, -15.4864) -> (-31.7305, -58)
  line L207 (-27.5, -53.7451) -> (-69.7695, -11.2315)
  line L208 (-74, -53.7451) -> (-31.7305, -11.2315)
  line L209 (-27.5, -15.4864) -> (-69.7695, -58)
  circle A121 centre (0, 27.625) radius 1.2295
  line L210 (0, 57.55) -> (0, 27.625)
  line L211 (74, -11.2315) -> (27.5, -58) construction
  line L212 (27.5, -11.2315) -> (74, -58) construction
  line L213 (74, -15.4864) -> (31.7305, -58)
  line L214 (27.5, -53.7451) -> (69.7695, -11.2315)
  line L215 (74, -53.7451) -> (31.7305, -11.2315)
  line L216 (27.5, -15.4864) -> (69.7695, -58)
  line L217 (-74, -30.8889) -> (-27.5, -30.8889)
  line L218 (-27.5, -30.8889) -> (-27.5, -37.6649)
  line L219 (-27.5, -37.6649) -> (-74, -37.6649)
  line L220 (-74, -37.6649) -> (-74, -30.8889)
  line L221 (74, -29.8889) -> (27.5, -29.8889)
  line L222 (27.5, -29.8889) -> (27.5, -37.6649)
  line L223 (27.5, -37.6649) -> (74, -37.6649)
  line L224 (74, -37.6649) -> (74, -29.8889)
  line L225 (-17.5, -11.2315) -> (18.5, -58)
  line L226 (-17.5, -58) -> (18.5, -11.2315)
  line L227 (-14.3451, -11.2315) -> (18.5, -53.9014)
  line L228 (-17.5, -53.9014) -> (15.3451, -11.2315)
  line L229 (-14.3451, -58) -> (18.5, -15.3301)
  line L230 (15.3451, -58) -> (-17.5, -15.3301)
  line L231 (-55.75, 6.7685) -> (-45.75, 6.7685)
  line L232 (-45.75, 6.7685) -> (-45.75, -3.2315)
  line L233 (-45.75, -3.2315) -> (-55.75, -3.2315)
  line L234 (-55.75, -3.2315) -> (-55.75, 6.7685)
  line L235 (-4.5, 6.7685) -> (5.5, 6.7685)
  line L236 (5.5, 6.7685) -> (5.5, -3.2315)
  line L237 (5.5, -3.2315) -> (-4.5, -3.2315)
  line L238 (-4.5, -3.2315) -> (-4.5, 6.7685)
  line L239 (45.75, 6.7685) -> (55.75, 6.7685)
  line L240 (55.75, 6.7685) -> (55.75, -3.2315)
  line L241 (55.75, -3.2315) -> (45.75, -3.2315)
  line L242 (45.75, -3.2315) -> (45.75, 6.7685)
  point P0 (0, 0)
  point P1 (74, -3.2315)
  point P2 (27.5, 6.7685)
  point P3 (11.6433, -3.2315)
  point P4 (11.6433, 6.7685)
  point P5 (-9.0142, 6.7685)
  point P6 (-17.5, -3.75)
  point P7 (-27.5, -3.2315)
  point P8 (-27.5, -3.75)
  point P9 (-74, -3.75)
  point P10 (43.4878, -37.6649)
  point P11 (27.5, -53.7451)
  point P12 (53.5282, -41.6649)
  point P13 (47.9718, -41.6649)
  point P14 (31.7305, -58)
  point P15 (69.7695, -58)
  point P16 (71.6586, -51.3901)
  point P17 (74, -51.3901)
  point P18 (74, -41.6649)
  point P19 (61.9892, -41.6649)
  point P20 (74, -15.4864)
  point P21 (59.6802, -29.8889)
  point P22 (51.2192, -29.8889)
  point P23 (69.7695, -11.2315)
  point P24 (31.7305, -11.2315)
  point P25 (50.2808, -29.8889)
  point P26 (27.5, -29.8889)
  point P27 (41.8198, -29.8889)
  point P28 (27.5, -15.4864)
  point P29 (0.5, -30.5172)
  point P30 (3.6549, -34.6158)
  point P31 (0.5, -38.7143)
  point P32 (-2.6549, -34.6158)
  point P33 (-43.4878, -37.6649)
  point P34 (-41.8198, -29.8889)
  point P35 (-50.2808, -29.8889)
  point P36 (-51.2192, -29.8889)
  point P37 (-58.6859, -30.8889)
  point P38 (-61.9892, -41.6649)
  point P39 (-74, -41.6649)
  point P40 (-50.75, -38.8707)
  point P41 (-27.5, 11.25)
  point P42 (-17.5, 11.25)
  point P43 (18.5, 11.25)
  point P44 (18.5, -8.75)
  point P45 (-17.5, -3.75)
  point P46 (-9.0142, -3.2315)
  point P47 (-74, 11.25)
  point P48 (-74, -3.75)
  point P49 (-27.5, -3.75)
  point P50 (41.4928, -39.6715)
  point P51 (67, -46.7047)
  point P52 (50.75, -30.3608)
  point P53 (-50.75, -30.3608)
  point P54 (-55.2521, -34.8889)
  point P55 (-42.4985, -38.66)
  point P56 (-67, -46.7047)
  point P57 (-74, -42.9318)
  point P58 (86, 37.9935)
  point P59 (86, 40.0065)
  point P60 (86, 15.2435)
  point P61 (86, 17.2565)
  point P62 (50.75, -38.8707)
  point P63 (74, -53.7451)
  point P64 (54.9805, -34.6158)
  point P65 (18.5, -3.2315)
  point P66 (5.5, 6.7685)
  point P67 (-4.5, -3.2315)
  point P68 (-47.9718, -41.6649)
  point P69 (-53.5282, -41.6649)
  point P70 (-39, -30.8889)
  point P71 (-42.8141, -30.8889)
  point P72 (-49.5512, -37.6649)
  point P73 (-46, -40.6649)
  point P74 (-52, -30.8889)
  point P75 (-74, -34.8889)
  point P76 (58.0122, -37.6649)
  point P77 (-58.0122, -37.6649)
  dimension "d108" = 5
  dimension "d110" = 0
  dimension "d111" = 0
  dimension "d114" = 0
  dimension "d115" = 0
  dimension "d118" = 8
  dimension "d119" = 10
  dimension "d120" = 3
  dimension "d121" = 3
  dimension "d122" = 6
  dimension "d124" = 6
  dimension "d125" = 3
  dimension "d126" = 2.5
  dimension "d127" = 5
  dimension "d128" = 5
  dimension "d129" = 2.5
  dimension "d132" = 5
  dimension "d133" = 10
  dimension "d134" = 10
  dimension "d135" = 10
  dimension "d136" = 18.25
  dimension "d137" = 18.25
  dimension "d138" = 13
  dimension "d139" = 13
  dimension "d140" = 18.25
  dimension "d141" = 18.25
  dimension "d144" = 4
  dimension "d145" = 1
  constraints: 170 end point, 51 point on line, 38 parallel, 18 horizontal, 14 perpendicular, 9 collinear, 8 symmetric about line, 4 vertical alignment, 1 tangent, 6 other
  measures "d108" distance between parallel lines of L160 L162
  measures "d110" distance between parallel lines of L178 L2
  measures "d111" distance between parallel lines of L4 L176
  measures "d114" distance between parallel lines of L180 L8
  measures "d115" distance between parallel lines of L182 L10
  measures "d118" distance between parallel lines of L192 L194
  measures "d119" distance between parallel lines of L184 L192
  measures "d120" distance between parallel lines of L204 L207
  measures "d121" distance between parallel lines of L204 L206
  measures "d122" distance between parallel lines of L206 L207
  measures "d124" distance between parallel lines of L208 L209
  measures "d125" distance between parallel lines of L205 L209
  measures "d126" distance between parallel lines of L225 L230
  measures "d127" distance between parallel lines of L230 L227
  measures "d128" distance between parallel lines of L229 L228
  measures "d129" distance between parallel lines of L226 L229
  measures "d132" distance between parallel lines of L174 L184
  measures "d133" distance between parallel lines of L234 L232
  measures "d134" distance between parallel lines of L238 L236
  measures "d135" distance between parallel lines of L240 L242
  measures "d136" distance between parallel lines of L232 L178
  measures "d137" distance between parallel lines of L164 L234
  measures "d138" distance between parallel lines of L236 L180
  measures "d139" distance between parallel lines of L238 L176
  measures "d140" distance between parallel lines of L240 L168
  measures "d141" distance between parallel lines of L182 L242
  measures "d144" distance between parallel lines of L219 L81
  measures "d145" distance between parallel lines of L89 L217
extrude "Extrusion4" cut sketch "Sketch10" against normal blind 10 contours L178 L217 L84 L85 L209 L2 | L85 L84 L217 L209 | L178 L18 L207 L83 L84 L219 | L208 L207 L85 | L85 L207 L194 L208 | L84 L83 L207 L219 | L230 L6 L5 L4 | L5 L6 L230 L228 L176 | L198 L228 L6 L227 | L192 L232 L184 L178 | L160 L209 L98 L99 L94 L206 | L176 L187 L135 L196 | L6 L228 L227 | L164 L184 L234 L192 | L206 L81 L209 | L94 L99 L98 L209 L81 L206 | L135 L187 L238 L196 | L206 L217 L164 | L208 L81 L164 L219 | L229 L230 L160 | L208 L79 L80 L164 L81 | L16 L182 L223 L56 L57 L214 | L213 L100 L101 L102 L216 L160 | L236 L187 L133 L196 | L8 L7 L6 L229 | L196 L133 L187 L180 | L6 L7 L180 L227 L229 | L208 L98 L164 L80 L79 | L57 L56 L223 L214 | L213 L59 L216 L102 L101 L100 | L164 L98 L208 | L216 L55 L221 L182 L10 | L182 L190 L242 L200 | L213 L216 L59 | L202 L214 L55 L215 | L200 L240 L190 L168 | L55 L214 L215 | L168 L55 L213 | L215 L102 L168 | L215 L59 L168 L60 L61 | L61 L60 L168 L102 L215 | L215 L223 L168 L59 | A37 | S2 L106 S3 L107 | L112 S5 L113 S4
fillet "Fillet6" radius 3 44 edges at (-74, 1.5, 6.7685) (-55.75, 1.5, 6.7685) (-74, 1.5, -3.2315) (-55.75, 1.5, -3.2315) (-45.75, 1.5, 6.7685) (-45.75, 1.5, -3.2315) (-27.5, 1.5, -3.2315) (-27.5, 1.5, 6.7685) (-17.5, 1.5, 6.7685) (-17.5, 1.5, -3.2315) (-4.5, 1.5, -3.2315) (-4.5, 1.5, 6.7685) (5.5, 1.5, 6.7685) (18.5, 1.5, -3.2315) (5.5, 1.5, -3.2315) (18.5, 1.5, 6.7685) (45.75, 1.5, 6.7685) (74, 1.5, 6.7685) (27.5, 1.5, -3.2315) (55.75, 1.5, -3.2315) (55.75, 1.5, 6.7685) (27.5, 1.5, 6.7685) (45.75, 1.5, -3.2315) (74, 1.5, -3.2315) (-31.7305, 1.5, -11.2315) (-69.7695, 1.5, -11.2315) (-50.75, 1.5, -30.3608) (-31.7305, 1.5, -58) (-69.7695, 1.5, -58) (-27.5, 1.5, -53.7451) (-27.5, 1.5, -37.6649) (-43.4878, 1.5, -37.6649) (-74, 1.5, -53.7451) (-74, 1.5, -15.4864) (-74, 1.5, -30.8889) (-58.6859, 1.5, -30.8889) (-27.5, 1.5, -30.8889) (18.5, 1.5, -53.9014) (-17.5, 1.5, -53.9014) (-17.5, 1.5, -15.3301) (15.3451, 1.5, -11.2315) (18.5, 1.5, -15.3301) (0.5, 1.5, -30.5172) (-14.3451, 1.5, -11.2315)
fillet "Fillet7" radius 3 26 edges at (0.5, 1.5, -38.7143) (15.3451, 1.5, -58) (-14.3451, 1.5, -58) (31.7305, 1.5, -58) (69.7695, 1.5, -58) (43.4878, 1.5, -37.6649) (27.5, 1.5, -53.7451) (27.5, 1.5, -37.6649) (74, 1.5, -53.7451) (74, 1.5, -15.4864) (74, 1.5, -29.8889) (59.6802, 1.5, -29.8889) (69.7695, 1.5, -11.2315) (50.75, 1.5, -30.3608) (31.7305, 1.5, -11.2315) (27.5, 1.5, -15.4864) (41.8198, 1.5, -29.8889) (27.5, 1.5, -29.8889) (74, 1.5, -37.6649) (58.0122, 1.5, -37.6649) (-50.75, 1.5, -38.8707) (50.75, 1.5, -38.8707) (-27.5, 1.5, -15.4864) (-42.8141, 1.5, -30.8889) (-58.0122, 1.5, -37.6649) (-74, 1.5, -37.6649)
equation "\"d11\" = d13"
body "Solid2"
